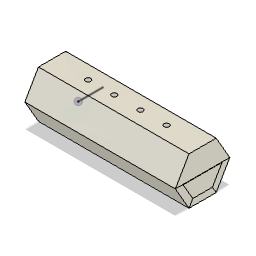
Ares_Pedroli_Dye—Radio (Autodesk Fusion 360 design; units mm, degrees)
Autodesk Fusion 360 part; units mm, degrees
note: some values were not read from the file. Set by a fixed rule: which sketch regions a step uses.
(part 1 of 3)
sketch "Schizzo1" plane through (0, 0, 0) normal (1, 0, 0) x (0, 0, -1)
  line L0 (20.7846, 36) -> (-20.7846, 36)
  line L1 (15.0111, 26) -> (-15.0111, 26)
  line L2 (-15.0111, 26) -> (-20.7846, 36)
  line L3 (15.0111, 26) -> (20.7846, 36)
  dimension "d1" = 36
  dimension "d2" = 26
  measures "d1" distance of origin L0
  measures "d2" distance of origin L1
extrude "Estrusione1" add sketch "Schizzo1" along normal blind 230 contours L0 L1 L2 L3 picked at (5.0037, 32.6667) makes body 1
sketch "Schizzo2" plane through (230, 0, 0) normal (1, 0, 0) x (0, 0, -1)
  line L0 (-15.0111, 26) -> (15.0111, 26)
  line L1 (15.0111, 26) -> (20.7846, 36)
  line L2 (20.7846, 36) -> (-20.7846, 36)
  line L3 (-20.7846, 36) -> (-15.0111, 26)
  line L4 (-15.0111, 26) -> (-20.7846, 36)
  line L5 (-20.7846, 36) -> (-41.5692, 0)
  line L6 (-41.5692, 0) -> (-30.0222, 0)
  line L7 (-30.0222, 0) -> (-15.0111, 26)
  line L8 (-30.0222, 0) -> (-41.5692, 0)
  line L9 (-41.5692, 0) -> (-20.7846, -36)
  line L10 (-20.7846, -36) -> (-15.0111, -26)
  line L11 (-15.0111, -26) -> (-30.0222, 0)
  line L12 (-15.0111, -26) -> (-20.7846, -36)
  line L13 (-20.7846, -36) -> (20.7846, -36)
  line L14 (20.7846, -36) -> (15.0111, -26)
  line L15 (15.0111, -26) -> (-15.0111, -26)
  line L16 (15.0111, -26) -> (20.7846, -36)
  line L17 (20.7846, -36) -> (41.5692, 0)
  line L18 (41.5692, 0) -> (30.0222, 0)
  line L19 (30.0222, 0) -> (15.0111, -26)
  line L20 (30.0222, 0) -> (41.5692, 0)
  line L21 (41.5692, 0) -> (20.7846, 36)
  line L22 (20.7846, 36) -> (15.0111, 26)
  line L23 (15.0111, 26) -> (30.0222, 0)
  dimension "d6" = 360
sketch "Schizzo3" plane through (230, 0, 0) normal (1, 0, 0) x (0, 0, -1)
extrude "Estrusione2" add sketch "Schizzo2" against normal blind 230 separate body contours L3 L4 L5 L6 L7 L8 picked at (-25.7883, 20.6667) makes body 2
sketch "Schizzo4" plane through (230, 0, 0) normal (1, 0, 0) x (0, 0, -1)
  line L0 (-15.0111, 26) -> (15.0111, 26)
  line L1 (15.0111, 26) -> (20.7846, 36)
  line L2 (20.7846, 36) -> (-20.7846, 36)
  line L3 (-20.7846, 36) -> (-15.0111, 26)
  line L4 (-20.7846, 36) -> (-41.5692, 0)
  line L5 (-41.5692, 0) -> (-20.7846, -36)
  line L6 (-20.7846, -36) -> (20.7846, -36)
  line L7 (20.7846, -36) -> (41.5692, 0)
  line L8 (41.5692, 0) -> (20.7846, 36)
  line L9 (20.7846, 36) -> (-20.7846, 36)
  line L10 (-15.0111, 26) -> (-30.0222, 0)
  line L11 (-30.0222, 0) -> (-15.0111, -26)
  line L12 (-15.0111, -26) -> (15.0111, -26)
  line L13 (15.0111, -26) -> (30.0222, 0)
  line L14 (30.0222, 0) -> (15.0111, 26)
  line L15 (15.0111, 26) -> (-15.0111, 26)
  line L16 (-15.0111, -26) -> (-20.7846, -36)
  line L17 (15.0111, -26) -> (20.7846, -36)
  dimension "d9" = 36
  dimension "d10" = 26
  measures "d9" distance of origin L9
  measures "d10" distance of origin L15
extrude "Estrusione3" add sketch "Schizzo4" against normal blind 230 separate body contours L6 L12 L16 L17 picked at (5.0037, -32.6667) makes body 3
sketch "Schizzo5" plane through (230, 0, 0) normal (1, 0, 0) x (0, 0, -1)
  line L0 (-15.0111, 26) -> (-20.7846, 36)
  line L1 (-20.7846, 36) -> (-41.5692, 0)
  line L2 (-41.5692, 0) -> (-30.0222, 0)
  line L3 (-30.0222, 0) -> (-15.0111, 26)
  line L4 (-20.7846, 36) -> (-41.5692, 0)
  line L5 (-41.5692, 0) -> (-20.7846, -36)
  line L6 (-20.7846, -36) -> (20.7846, -36)
  line L7 (20.7846, -36) -> (41.5692, 0)
  line L8 (41.5692, 0) -> (20.7846, 36)
  line L9 (20.7846, 36) -> (-20.7846, 36)
  line L10 (-15.0111, 26) -> (-30.0222, 0)
  line L11 (-30.0222, 0) -> (-15.0111, -26)
  line L12 (-15.0111, -26) -> (15.0111, -26)
  line L13 (15.0111, -26) -> (30.0222, 0)
  line L14 (30.0222, 0) -> (15.0111, 26)
  line L15 (15.0111, 26) -> (-15.0111, 26)
  line L16 (15.0111, -26) -> (20.7846, -36)
  line L17 (30.0222, 0) -> (41.5692, 0)
  dimension "d13" = 36
  dimension "d14" = 26
  constraint horizontal L17
  measures "d13" distance of origin L9
  measures "d14" distance of origin L15
extrude "Estrusione4" add sketch "Schizzo5" against normal blind 230 separate body contours L7 L13 L16 L17 picked at (25.7883, -20.6667) makes body 4
sketch "Schizzo6" plane through (230, 0, 0) normal (1, 0, 0) x (0, 0, -1)
  line L0 (-15.0111, 26) -> (15.0111, 26)
  line L1 (15.0111, 26) -> (20.7846, 36)
  line L2 (20.7846, 36) -> (-20.7846, 36)
  line L3 (-20.7846, 36) -> (-15.0111, 26)
  line L4 (-20.7846, 36) -> (-41.5692, 0)
  line L5 (-41.5692, 0) -> (-20.7846, -36)
  line L6 (-20.7846, -36) -> (20.7846, -36)
  line L7 (20.7846, -36) -> (41.5692, 0)
  line L8 (41.5692, 0) -> (20.7846, 36)
  line L9 (20.7846, 36) -> (-20.7846, 36)
  line L10 (-15.0111, 26) -> (-30.0222, 0)
  line L11 (-30.0222, 0) -> (-15.0111, -26)
  line L12 (-15.0111, -26) -> (15.0111, -26)
  line L13 (15.0111, -26) -> (30.0222, 0)
  line L14 (30.0222, 0) -> (15.0111, 26)
  line L15 (15.0111, 26) -> (-15.0111, 26)
  line L16 (-30.0222, 0) -> (-41.5692, 0)
  line L17 (-15.0111, -26) -> (-20.7846, -36)
  dimension "d17" = 36
  dimension "d18" = 26
  constraint horizontal L16
  measures "d17" distance of origin L9
  measures "d18" distance of origin L15
extrude "Estrusione5" add sketch "Schizzo6" against normal blind 230 separate body contours L5 L11 L16 L17 picked at (-25.7883, -20.6667) makes body 5
sketch "Schizzo7" plane through (230, 0, 0) normal (1, 0, 0) x (0, 0, -1)
  line L0 (-15.0111, 26) -> (15.0111, 26)
  line L1 (15.0111, 26) -> (20.7846, 36)
  line L2 (20.7846, 36) -> (-20.7846, 36)
  line L3 (-20.7846, 36) -> (-15.0111, 26)
  line L4 (-20.7846, 36) -> (-41.5692, 0)
  line L5 (-41.5692, 0) -> (-20.7846, -36)
  line L6 (-20.7846, -36) -> (20.7846, -36)
  line L7 (20.7846, -36) -> (41.5692, 0)
  line L8 (41.5692, 0) -> (20.7846, 36)
  line L9 (20.7846, 36) -> (-20.7846, 36)
  line L10 (-15.0111, 26) -> (-30.0222, 0)
  line L11 (-30.0222, 0) -> (-15.0111, -26)
  line L12 (-15.0111, -26) -> (15.0111, -26)
  line L13 (15.0111, -26) -> (30.0222, 0)
  line L14 (30.0222, 0) -> (15.0111, 26)
  line L15 (15.0111, 26) -> (-15.0111, 26)
  line L16 (30.0222, 0) -> (41.5692, 0)
  line L17 (15.0111, 26) -> (20.7846, 36)
  dimension "d21" = 36
  dimension "d22" = 26
  constraint horizontal L16
  constraint coincident L0.end L1.start
  constraint coincident L1.end L2.start
  measures "d21" distance of origin L9
  measures "d22" distance of origin L15
extrude "Estrusione6" add sketch "Schizzo7" against normal blind 230 separate body contours L1 L8 L14 L16 L17 picked at (25.7883, 20.6667) makes body 6
sketch "Schizzo8" plane through (0, 0, 0) normal (0, -0.5, -0.866025) x (-1, 0, 0)
  line L0 (0, 30.0222) -> (0, 41.5692)
  line L1 (0, 41.5692) -> (-230, 41.5692)
  line L2 (-230, 41.5692) -> (-230, 30.0222)
  line L3 (-230, 30.0222) -> (0, 30.0222)
sketch "Schizzo9" plane through (0, 0, 0) normal (0, -0.5, -0.866025) x (-1, 0, 0)
sketch "Schizzo10" plane through (0, 0, 0) normal (0, 0, 1) x (1, 0, 0)
sketch "Schizzo11" plane through (0, 0, 0) normal (0, 0, 1) x (1, 0, 0)
ref_plane "Piano di lavoro1" through (0, 0, -50) normal (0, 0, 1) x (1, 0, 0)
sketch "Schizzo12" plane through (0, 0, -50) normal (0, 0, 1) x (1, 0, 0)
sketch "Schizzo13" plane through (0, 0, 0) normal (1, 0, 0) x (0, 0, -1)
  line L0 (-20.7846, 36) -> (-41.5692, 0)
  line L1 (-41.5692, 0) -> (-20.7846, -36)
  line L2 (-20.7846, -36) -> (20.7846, -36)
  line L3 (20.7846, -36) -> (41.5692, 0)
  line L4 (41.5692, 0) -> (20.7846, 36)
  line L5 (20.7846, 36) -> (-20.7846, 36)
  dimension "d26" = 36
  measures "d26" distance of origin L5
ref_plane "Piano di lavoro2" through (10, 0, 0) normal (1, 0, 0) x (0, 0, -1)
sketch "Schizzo14" plane through (10, 0, 0) normal (1, 0, 0) x (0, 0, -1)
  line L0 (-15.0111, 26) -> (-30.0222, 0)
  line L1 (-30.0222, 0) -> (-15.0111, -26)
  line L2 (-15.0111, -26) -> (15.0111, -26)
  line L3 (15.0111, -26) -> (30.0222, 0)
  line L4 (30.0222, 0) -> (15.0111, 26)
  line L5 (15.0111, 26) -> (-15.0111, 26)
  dimension "d28" = 26
  measures "d28" distance of origin L5
loft "Loft1" add profiles "Schizzo13", "Schizzo14" section 1 contours L0 L1 L2 L3 L4 L5 picked at (-6.9282, -12) section 2 contours L0 L1 L2 L3 L4 L5 picked at (5.0037, 8.6667) separate body makes body 7
ref_plane "Piano di lavoro3" through (0, 36, 0) normal (0.707107, 0.707107, 0) x (0, 0, 1)
sketch "Schizzo15" plane through (18, 18, 0) normal (0.707107, 0.707107, 0) x (0, 0, 1)
  line L0 (-25.4045, -30.5953) -> (26.5037, -30.5953)
  line L1 (26.5037, -30.5953) -> (26.5037, -11.2977)
  line L2 (26.5037, -11.2977) -> (-25.4045, -11.2977)
  line L3 (-25.4045, -11.2977) -> (-25.4045, -30.5953)
  constraint horizontal L0
  constraint vertical L1
  constraint horizontal L2
  constraint vertical L3
extrude "Estrusione7" cut sketch "Schizzo15" against normal blind 9 contours L0 L1 L2 L3 picked at (9.201, -24.1628) bodies 1
ref_plane "Piano di lavoro4" through (0, -36, 0) normal (-0.707107, 0.707107, 0) x (0, 0, 1)
sketch "Schizzo17" plane through (18, -18, 0) normal (-0.707107, 0.707107, 0) x (0, 0, 1)
  line L0 (-27.9444, 2.5294) -> (34.6896, 2.5294)
  line L1 (34.6896, 2.5294) -> (34.6896, -37.219)
  line L2 (34.6896, -37.219) -> (-27.9444, -37.219)
  line L3 (-27.9444, -37.219) -> (-27.9444, 2.5294)
  constraint horizontal L0
  constraint vertical L1
  constraint horizontal L2
  constraint vertical L3
sketch "Schizzo18" plane through (18, -18, 0) normal (-0.707107, 0.707107, 0) x (0, 0, 1)
extrude "Estrusione8" cut sketch "Schizzo17" along normal blind 15 contours L0 L1 L2 L3 picked at (-7.0664, -10.72) bodies 3
ref_plane "Piano di lavoro5" through (0, 18, -31.1769) normal (0.707107, 0.353553, -0.612372) x (0, -0.866025, -0.5)
sketch "Schizzo19" plane through (18, 9, -15.5885) normal (0.707107, 0.353553, -0.612372) x (0, -0.866025, -0.5)
  line L0 (28.5212, 30.9976) -> (-31.4246, 30.9976)
  line L1 (-31.4246, 30.9976) -> (-31.4246, 0.2562)
  line L2 (-31.4246, 0.2562) -> (28.5212, 0.2562)
  line L3 (28.5212, 0.2562) -> (28.5212, 30.9976)
  constraint horizontal L0
  constraint vertical L1
  constraint horizontal L2
  constraint vertical L3
extrude "Estrusione9" cut sketch "Schizzo19" against normal blind 15 contours L0 L1 L2 L3 picked at (-11.4427, 10.5033) bodies 6
ref_plane "Piano di lavoro6" through (0, -18, 31.1769) normal (0.707107, -0.353553, 0.612372) x (0, 0.866025, 0.5)
sketch "Schizzo20" plane through (18, -9, 15.5885) normal (0.707107, -0.353553, 0.612372) x (0, 0.866025, 0.5)
  line L0 (-39.5033, -4.678) -> (44.909, -4.678)
  line L1 (44.909, -4.678) -> (44.909, 45.013)
  line L2 (44.909, 45.013) -> (-39.5033, 45.013)
  line L3 (-39.5033, 45.013) -> (-39.5033, -4.678)
  constraint horizontal L0
  constraint vertical L1
  constraint horizontal L2
  constraint vertical L3
extrude "Estrusione10" cut sketch "Schizzo20" against normal blind 15 contours L0 L1 L2 L3 picked at (-11.3659, 28.4493) bodies 5
ref_plane "Piano di lavoro7" through (0, 13, 22.5167) normal (0.707107, -0.353553, -0.612372) x (0, -0.866025, 0.5)
sketch "Schizzo21" plane through (-13, 6.5, 11.2583) normal (0.707107, -0.353553, -0.612372) x (0, -0.866025, 0.5)
ref_plane "Piano di lavoro8" through (0, 18, 31.1769) normal (0.707107, 0.353553, 0.612372) x (0, 0.866025, -0.5)
sketch "Schizzo22" plane through (18, 9, 15.5885) normal (0.707107, 0.353553, 0.612372) x (0, 0.866025, -0.5)
  line L0 (34.112, 42.0471) -> (-37.7603, 42.0471)
  line L1 (-37.7603, 42.0471) -> (-37.7603, -13.0428)
  line L2 (-37.7603, -13.0428) -> (34.112, -13.0428)
  line L3 (34.112, -13.0428) -> (34.112, 42.0471)
  constraint horizontal L0
  constraint vertical L1
  constraint horizontal L2
  constraint vertical L3
extrude "Estrusione11" cut sketch "Schizzo22" against normal blind 15 contours L0 L1 L2 L3 picked at (-13.8029, 23.6838) bodies 2
ref_plane "Piano di lavoro9" through (0, -18, -31.1769) normal (0.707107, -0.353553, -0.612372) x (0, -0.866025, 0.5)
sketch "Schizzo23" plane through (18, -9, -15.5885) normal (0.707107, -0.353553, -0.612372) x (0, -0.866025, 0.5)
  line L0 (-34.6034, -9.0564) -> (39.4695, -9.0564)
  line L1 (39.4695, -9.0564) -> (39.4695, 34.7386)
  line L2 (39.4695, 34.7386) -> (-34.6034, 34.7386)
  line L3 (-34.6034, 34.7386) -> (-34.6034, -9.0564)
  constraint horizontal L0
  constraint vertical L1
  constraint horizontal L2
  constraint vertical L3
extrude "Estrusione12" cut sketch "Schizzo23" against normal blind 30 contours L0 L1 L2 L3 picked at (14.7785, 20.1402) bodies 4
sketch "Schizzo24" plane through (230, 0, 0) normal (1, 0, 0) x (0, 0, -1)
  line L0 (-15.0111, 26) -> (15.0111, 26)
  line L1 (15.0111, 26) -> (20.7846, 36)
  line L2 (20.7846, 36) -> (-20.7846, 36)
  line L3 (-20.7846, 36) -> (-15.0111, 26)
  line L4 (-20.7846, 36) -> (-41.5692, 0)
  line L5 (-41.5692, 0) -> (-20.7846, -36)
  line L6 (-20.7846, -36) -> (20.7846, -36)
  line L7 (20.7846, -36) -> (41.5692, 0)
  line L8 (41.5692, 0) -> (20.7846, 36)
  line L9 (20.7846, 36) -> (-20.7846, 36)
  dimension "d48" = 36
  measures "d48" distance of origin L9
ref_plane "Piano di lavoro10" through (220, 0, 0) normal (1, 0, 0) x (0, 0, -1)
sketch "Schizzo25" plane through (220, 0, 0) normal (1, 0, 0) x (0, 0, -1)
  line L0 (-15.0111, 26) -> (-30.0222, 0)
  line L1 (-30.0222, 0) -> (-15.0111, -26)
  line L2 (-15.0111, -26) -> (15.0111, -26)
  line L3 (15.0111, -26) -> (30.0222, 0)
  line L4 (30.0222, 0) -> (15.0111, 26)
  line L5 (15.0111, 26) -> (-15.0111, 26)
  dimension "d50" = 26
  measures "d50" distance of origin L5
loft "Loft2" add profiles "Schizzo24", "Schizzo25" section 1 contours L0 L1 L2 L3 L9 | L0 L1 L3 L4 L5 L6 L7 L8 picked at (5.0037, 32.6667) picked at (5.0037, -15.3333) section 2 contours L0 L1 L2 L3 L4 L5 picked at (5.0037, 8.6667) separate body makes body 8
sketch "Schizzo26" plane through (230, 0, 0) normal (1, 0, 0) x (0, 0, -1)
  line L0 (-15.0111, 26) -> (15.0111, 26)
  line L1 (15.0111, 26) -> (20.7846, 36)
  line L2 (20.7846, 36) -> (-20.7846, 36)
  line L3 (-20.7846, 36) -> (-15.0111, 26)
ref_plane "Piano di lavoro11" through (230, 31, 0) normal (1, 0, 0) x (0, 0, -1)
ref_plane "Piano di lavoro12" through (230, 18, 31.1769) normal (0.707107, -0.353553, -0.612372) x (0, -0.866025, 0.5)
sketch "Schizzo27" plane through (97, -48.5, -84.0045) normal (0.707107, -0.353553, -0.612372) x (0, -0.866025, 0.5)
  line L0 (22.2001, -191.6814) -> (-22.8191, -191.6814)
  line L1 (-22.8191, -191.6814) -> (-22.8191, -156.9019)
  line L2 (-22.8191, -156.9019) -> (22.2001, -156.9019)
  line L3 (22.2001, -156.9019) -> (22.2001, -191.6814)
  constraint horizontal L0
  constraint vertical L1
  constraint horizontal L2
  constraint vertical L3
extrude "Estrusione13" cut sketch "Schizzo27" along normal blind 15 contours L0 L1 L2 L3 picked at (7.1937, -168.495) bodies 2
ref_plane "Piano di lavoro13" through (230, 36, 0) normal (-0.707107, 0.707107, 0) x (0, 0, 1)
sketch "Schizzo28" plane through (97, -97, 0) normal (-0.707107, 0.707107, 0) x (0, 0, 1)
  line L0 (24.2107, 192.65) -> (-25.7482, 192.65)
  line L1 (-25.7482, 192.65) -> (-25.7482, 160.1447)
  line L2 (-25.7482, 160.1447) -> (24.2107, 160.1447)
  line L3 (24.2107, 160.1447) -> (24.2107, 192.65)
  constraint horizontal L0
  constraint vertical L1
  constraint horizontal L2
  constraint vertical L3
extrude "Estrusione14" cut sketch "Schizzo28" against normal blind 15 contours L0 L1 L2 L3 picked at (-9.0953, 181.8149) bodies 1
ref_plane "Piano di lavoro14" through (230, 18, -31.1769) normal (0.707107, -0.353553, 0.612372) x (0, 0.866025, 0.5)
sketch "Schizzo29" plane through (97, -48.5, 84.0045) normal (0.707107, -0.353553, 0.612372) x (0, 0.866025, 0.5)
  line L0 (24.9926, -195.9491) -> (-24.9663, -195.9491)
  line L1 (-24.9663, -195.9491) -> (-24.9663, -159.7609)
  line L2 (-24.9663, -159.7609) -> (24.9926, -159.7609)
  line L3 (24.9926, -159.7609) -> (24.9926, -195.9491)
  constraint horizontal L0
  constraint vertical L1
  constraint horizontal L2
  constraint vertical L3
extrude "Estrusione15" cut sketch "Schizzo29" along normal blind 15 contours L0 L1 L2 L3 picked at (8.3396, -183.8864) bodies 6
sketch "Schizzo30" plane through (230, 0, 0) normal (1, 0, 0) x (0, 0, -1)
  line L0 (20.7846, 36) -> (-20.7846, 36)
  line L1 (-20.7846, 36) -> (-41.5692, 0)
  line L2 (-41.5692, 0) -> (-20.7846, -36)
  line L3 (-20.7846, -36) -> (20.7846, -36)
  line L4 (20.7846, -36) -> (41.5692, 0)
  line L5 (41.5692, 0) -> (20.7846, 36)
  line L6 (-51.0641, 0) -> (47.9858, 0)
  line L7 (47.9858, 0) -> (47.9858, -40.8332)
  line L8 (47.9858, -40.8332) -> (-51.0641, -40.8332)
  line L9 (-51.0641, -40.8332) -> (-51.0641, 0)
  constraint horizontal L6
  constraint vertical L7
  constraint horizontal L8
  constraint vertical L9
extrude "Estrusione16" cut sketch "Schizzo30" against normal blind 50 contours L2 L3 L4 L6 L7 L8 L9 | L2 L3 L4 L6 picked at (-37.806, -25.6111) picked at (-6.9282, -12) bodies 8
sketch "Schizzo31" plane through (0, 0, 0) normal (1, 0, 0) x (0, 0, -1)
ref_plane "Piano di lavoro15" through (230, 0, 0) normal (1, 0, 0) x (0, 1, 0)
sketch "Schizzo32" plane through (230, 0, 0) normal (1, 0, 0) x (0, 0, -1)
  line L0 (-15.0111, 26) -> (-30.0222, 0)
  line L1 (-30.0222, 0) -> (-15.0111, -26)
  line L2 (-15.0111, -26) -> (15.0111, -26)
  line L3 (15.0111, -26) -> (30.0222, 0)
  line L4 (30.0222, 0) -> (15.0111, 26)
  line L5 (15.0111, 26) -> (-15.0111, 26)
  line L6 (-12.1244, 21) -> (-24.2487, 0)
  line L7 (-24.2487, 0) -> (-12.1244, -21)
  line L8 (-12.1244, -21) -> (12.1244, -21)
  line L9 (12.1244, -21) -> (24.2487, 0)
  line L10 (24.2487, 0) -> (12.1244, 21)
  line L11 (12.1244, 21) -> (-12.1244, 21)
  line L12 (-24.2487, 0) -> (-30.0222, 0)
  line L13 (-12.1244, -21) -> (-15.0111, -26)
  dimension "d64" = 26
  dimension "d65" = 21
  constraint horizontal L12
  measures "d64" distance of origin L5
  measures "d65" distance of origin L11
extrude "Estrusione17" add sketch "Schizzo32" against normal blind 190 separate body contours L1 L7 L12 L13 picked at (-19.0526, -15.6667) makes body 9
sketch "Schizzo33" plane through (230, 0, 0) normal (1, 0, 0) x (0, 0, -1)
  line L0 (-24.2487, 0) -> (-30.0222, 0)
  line L1 (-30.0222, 0) -> (-15.0111, -26)
  line L2 (-15.0111, -26) -> (-12.1244, -21)
  line L3 (-12.1244, -21) -> (-24.2487, 0)
  line L4 (-15.0111, 26) -> (-30.0222, 0)
  line L5 (-30.0222, 0) -> (-15.0111, -26)
  line L6 (-15.0111, -26) -> (15.0111, -26)
  line L7 (15.0111, -26) -> (30.0222, 0)
  line L8 (30.0222, 0) -> (15.0111, 26)
  line L9 (15.0111, 26) -> (-15.0111, 26)
  line L10 (12.1244, -21) -> (24.2487, 0)
  line L11 (24.2487, 0) -> (12.1244, 21)
  line L12 (12.1244, 21) -> (-12.1244, 21)
  line L13 (-12.1244, 21) -> (-24.2487, 0)
  line L14 (-24.2487, 0) -> (-12.1244, -21)
  line L15 (-12.1244, -21) -> (12.1244, -21)
  line L16 (12.1244, -21) -> (15.0111, -26)
  line L17 (24.2487, 0) -> (30.0222, 0)
  dimension "d68" = 26
  dimension "d69" = 21
  constraint horizontal L17
  measures "d68" distance of origin L9
  measures "d69" distance of origin L15
extrude "Estrusione18" add sketch "Schizzo33" against normal blind 190 separate body contours L7 L10 L16 L17 picked at (19.0526, -15.6667) makes body 10
sketch "Schizzo34" plane through (230, 0, 0) normal (1, 0, 0) x (0, 0, -1)
  line L0 (-24.2487, 0) -> (-30.0222, 0)
  line L1 (-30.0222, 0) -> (-15.0111, -26)
  line L2 (-15.0111, -26) -> (-12.1244, -21)
  line L3 (-12.1244, -21) -> (-24.2487, 0)
  line L4 (-15.0111, 26) -> (-30.0222, 0)
  line L5 (-30.0222, 0) -> (-15.0111, -26)
  line L6 (-15.0111, -26) -> (15.0111, -26)
  line L7 (15.0111, -26) -> (30.0222, 0)
  line L8 (30.0222, 0) -> (15.0111, 26)
  line L9 (15.0111, 26) -> (-15.0111, 26)
  line L10 (12.1244, -21) -> (24.2487, 0)
  line L11 (24.2487, 0) -> (12.1244, 21)
  line L12 (12.1244, 21) -> (-12.1244, 21)
  line L13 (-12.1244, 21) -> (-24.2487, 0)
  line L14 (-24.2487, 0) -> (-12.1244, -21)
  line L15 (-12.1244, -21) -> (12.1244, -21)
  line L16 (-12.1244, -21) -> (-15.0111, -26)
  line L17 (12.1244, -21) -> (15.0111, -26)
  dimension "d72" = 26
  dimension "d73" = 21
  constraint coincident L2.end L3.start
  constraint parallel L2 L16
  measures "d72" distance of origin L9
  measures "d73" distance of origin L15
extrude "Estrusione19" add sketch "Schizzo34" against normal blind 190 separate body contours L2 L6 L15 L16 L17 picked at (4.0415, -24.3333) makes body 11
sketch "Schizzo35" plane through (230, 0, 0) normal (1, 0, 0) x (0, 0, -1)
  line L0 (-12.1244, -21) -> (-15.0111, -26)
  line L1 (-15.0111, -26) -> (15.0111, -26)
  line L2 (15.0111, -26) -> (12.1244, -21)
  line L3 (12.1244, -21) -> (-12.1244, -21)
  line L4 (-15.0111, 26) -> (-30.0222, 0)
  line L5 (-30.0222, 0) -> (-15.0111, -26)
  line L6 (-15.0111, -26) -> (15.0111, -26)
  line L7 (15.0111, -26) -> (30.0222, 0)
  line L8 (30.0222, 0) -> (15.0111, 26)
  line L9 (15.0111, 26) -> (-15.0111, 26)
  dimension "d76" = 26
  measures "d76" distance of origin L9
ref_plane "Piano di lavoro16" through (225, 0, 0) normal (1, 0, 0) x (0, 0, -1)
sketch "Schizzo36" plane through (230, 0, 0) normal (1, 0, 0) x (0, 0, -1)
  line L0 (-41.5692, 0) -> (41.5692, 0)
  line L1 (41.5692, 0) -> (20.7846, 36)
  line L2 (20.7846, 36) -> (-20.7846, 36)
  line L3 (-20.7846, 36) -> (-41.5692, 0)
  line L4 (-15.0111, 26) -> (-30.0222, 0)
  line L5 (-30.0222, 0) -> (-15.0111, -26)
  line L6 (-15.0111, -26) -> (15.0111, -26)
  line L7 (15.0111, -26) -> (30.0222, 0)
  line L8 (30.0222, 0) -> (15.0111, 26)
  line L9 (15.0111, 26) -> (-15.0111, 26)
  dimension "d78" = 26
  measures "d78" distance of origin L9
sketch "Schizzo37" plane through (225, 0, 0) normal (1, 0, 0) x (0, 0, -1)
  line L0 (-12.1244, 21) -> (-24.2487, 0)
  line L1 (-24.2487, 0) -> (-12.1244, -21)
  line L2 (-12.1244, -21) -> (12.1244, -21)
  line L3 (12.1244, -21) -> (24.2487, 0)
  line L4 (24.2487, 0) -> (12.1244, 21)
  line L5 (12.1244, 21) -> (-12.1244, 21)
  dimension "d79" = 21
  measures "d79" distance of origin L5
loft "Loft3" add profiles "Schizzo35", "Schizzo37" section 1 contours L0 L1 L2 L3 L6 | L0 L2 L3 L4 L5 L7 L8 L9 picked at (4.0415, -24.3333) picked at (-4.0415, 10.3333) section 2 contours L0 L1 L2 L3 L4 L5 picked at (4.0415, 7) separate body makes body 12
ref_plane "Piano di lavoro17" through (230, -26, 0) normal (0.707107, 0.707107, 0) x (0, 0, -1)
sketch "Schizzo38" plane through (102, 102, 0) normal (0.707107, 0.707107, 0) x (0, 0, -1)
  line L0 (-16.091, -182.4296) -> (16.5053, -182.4296)
  line L1 (16.5053, -182.4296) -> (16.5053, -162.3983)
  line L2 (16.5053, -162.3983) -> (-16.091, -162.3983)
  line L3 (-16.091, -162.3983) -> (-16.091, -182.4296)
  constraint horizontal L0
  constraint vertical L1
  constraint horizontal L2
  constraint vertical L3
extrude "Estrusione20" cut sketch "Schizzo38" along normal blind 6 contours L0 L1 L2 L3 picked at (-5.2256, -169.0754) bodies 11
ref_plane "Piano di lavoro18" through (230, -13, -22.5167) normal (0.707107, 0.353553, 0.612372) x (0, 0.866025, -0.5)
sketch "Schizzo39" plane through (102, 51, 88.3346) normal (0.707107, 0.353553, 0.612372) x (0, 0.866025, -0.5)
  line L0 (-15.7064, -182.521) -> (18.7477, -182.521)
  line L1 (18.7477, -182.521) -> (18.7477, -158.8555)
  line L2 (18.7477, -158.8555) -> (-15.7064, -158.8555)
  line L3 (-15.7064, -158.8555) -> (-15.7064, -182.521)
  constraint horizontal L0
  constraint vertical L1
  constraint horizontal L2
  constraint vertical L3
sketch "Schizzo40" plane through (102, 51, 88.3346) normal (0.707107, 0.353553, 0.612372) x (0, 0.866025, -0.5)
extrude "Estrusione21" cut sketch "Schizzo39" along normal blind 7 contours L0 L1 L2 L3 picked at (-4.2217, -174.6325) bodies 10
ref_plane "Piano di lavoro19" through (230, -13, 22.5167) normal (0.707107, 0.353553, -0.612372) x (0, -0.866025, -0.5)
sketch "Schizzo41" plane through (102, 51, -88.3346) normal (0.707107, 0.353553, -0.612372) x (0, -0.866025, -0.5)
  line L0 (-15.9646, -162.8849) -> (17.7885, -162.8849)
  line L1 (17.7885, -162.8849) -> (17.7885, -184.9057)
  line L2 (17.7885, -184.9057) -> (-15.9646, -184.9057)
  line L3 (-15.9646, -184.9057) -> (-15.9646, -162.8849)
  constraint horizontal L0
  constraint vertical L1
  constraint horizontal L2
  constraint vertical L3
extrude "Estrusione22" cut sketch "Schizzo41" along normal blind 5 contours L0 L1 L2 L3 picked at (-4.7135, -170.2252) bodies 9
sketch "Schizzo42" plane through (230, 0, 0) normal (1, 0, 0) x (0, 0, -1)
  line L0 (15.0111, 26) -> (-15.0111, 26)
  line L1 (-15.0111, 26) -> (-30.0222, 0)
  line L2 (-30.0222, 0) -> (-15.0111, -26)
  line L3 (-15.0111, -26) -> (15.0111, -26)
  line L4 (15.0111, -26) -> (30.0222, 0)
  line L5 (30.0222, 0) -> (15.0111, 26)
  line L6 (-35.3311, 0) -> (32.3333, 0)
  line L7 (32.3333, 0) -> (32.3333, 27.8901)
  line L8 (32.3333, 27.8901) -> (-35.3311, 27.8901)
  line L9 (-35.3311, 27.8901) -> (-35.3311, 0)
  constraint horizontal L6
  constraint vertical L7
  constraint horizontal L8
  constraint vertical L9
extrude "Estrusione23" cut sketch "Schizzo42" against normal blind 11 contours L0 L1 L5 L6 | L0 L1 L5 L6 L7 L8 L9 picked at (5.0037, 8.6667) picked at (-26.7881, 17.9634) bodies 12
ref_plane "Piano di lavoro20" through (40, -13, -22.5167) normal (0.707107, -0.353553, -0.612372) x (0, -0.866025, 0.5)
sketch "Schizzo43" plane through (33, -16.5, -28.5788) normal (0.707107, -0.353553, -0.612372) x (0, -0.866025, 0.5)
  line L0 (-15.7171, -8.5355) -> (17.9237, -8.5355)
  line L1 (17.9237, -8.5355) -> (17.9237, -25.9435)
  line L2 (17.9237, -25.9435) -> (-15.7171, -25.9435)
  line L3 (-15.7171, -25.9435) -> (-15.7171, -8.5355)
  constraint horizontal L0
  constraint vertical L1
  constraint horizontal L2
  constraint vertical L3
extrude "Estrusione24" cut sketch "Schizzo43" against normal blind 6 contours L0 L1 L2 L3 picked at (-4.5035, -14.3381) bodies 10
ref_plane "Piano di lavoro21" through (40, -26, 0) normal (-0.707107, 0.707107, 0) x (0, 0, 1)
sketch "Schizzo44" plane through (33, -33, 0) normal (-0.707107, 0.707107, 0) x (0, 0, 1)
  line L0 (-17.0445, 8.6761) -> (20.7303, 8.6761)
  line L1 (20.7303, 8.6761) -> (20.7303, 23.9726)
  line L2 (20.7303, 23.9726) -> (-17.0445, 23.9726)
  line L3 (-17.0445, 23.9726) -> (-17.0445, 8.6761)
  constraint horizontal L0
  constraint vertical L1
  constraint horizontal L2
  constraint vertical L3
extrude "Estrusione25" cut sketch "Schizzo44" along normal blind 8 contours L0 L1 L2 L3 picked at (-4.4529, 13.775) bodies 11
ref_plane "Piano di lavoro22" through (40, -13, 22.5167) normal (0.707107, -0.353553, 0.612372) x (0, 0.866025, 0.5)
sketch "Schizzo45" plane through (33, -16.5, 28.5788) normal (0.707107, -0.353553, 0.612372) x (0, 0.866025, 0.5)
  line L0 (-16.1058, -7.4381) -> (17.3139, -7.4381)
  line L1 (17.3139, -7.4381) -> (17.3139, -25.1355)
  line L2 (17.3139, -25.1355) -> (-16.1058, -25.1355)
  line L3 (-16.1058, -25.1355) -> (-16.1058, -7.4381)
  constraint horizontal L0
  constraint vertical L1
  constraint horizontal L2
  constraint vertical L3
extrude "Estrusione26" cut sketch "Schizzo45" against normal blind 7 contours L0 L1 L2 L3 picked at (-4.9659, -13.3372) bodies 9
ref_plane "Piano di lavoro23" through (40, 0, 0) normal (1, 0, 0) x (0, 1, 0)
sketch "Schizzo46" plane through (40, 0, 0) normal (1, 0, 0) x (0, 0, -1)
  line L0 (-15.0111, 26) -> (-30.0222, 0)
  line L1 (-30.0222, 0) -> (-15.0111, -26)
  line L2 (-15.0111, -26) -> (15.0111, -26)
  line L3 (15.0111, -26) -> (30.0222, 0)
  line L4 (30.0222, 0) -> (15.0111, 26)
  line L5 (15.0111, 26) -> (-15.0111, 26)
  dimension "d101" = 26
  measures "d101" distance of origin L5
ref_plane "Piano di lavoro24" through (45, 0, 0) normal (1, 0, 0) x (0, 0, -1)
sketch "Schizzo47" plane through (45, 0, 0) normal (1, 0, 0) x (0, 0, -1)
  line L0 (-12.1244, 21) -> (-24.2487, 0)
  line L1 (-24.2487, 0) -> (-12.1244, -21)
  line L2 (-12.1244, -21) -> (12.1244, -21)
  line L3 (12.1244, -21) -> (24.2487, 0)
  line L4 (24.2487, 0) -> (12.1244, 21)
  line L5 (12.1244, 21) -> (-12.1244, 21)
  dimension "d103" = 21
  measures "d103" distance of origin L5
loft "Loft4" add profiles "Schizzo46", "Schizzo47" section 1 contours L0 L1 L2 L3 L4 L5 picked at (-5.0037, -8.6667) section 2 contours L0 L1 L2 L3 L4 L5 picked at (-4.0415, 7) separate body makes body 13
sketch "Schizzo48" plane through (40, 0, 0) normal (-1, 0, 0) x (0, 0, 1)
  line L0 (15.0111, 26) -> (-15.0111, 26)
  line L1 (-15.0111, 26) -> (-30.0222, 0)
  line L2 (-30.0222, 0) -> (-15.0111, -26)
  line L3 (-15.0111, -26) -> (15.0111, -26)
  line L4 (15.0111, -26) -> (30.0222, 0)
  line L5 (30.0222, 0) -> (15.0111, 26)
  line L6 (-38.2161, 0) -> (38.5243, 0)
  line L7 (38.5243, 0) -> (38.5243, 31.2047)
  line L8 (38.5243, 31.2047) -> (-38.2161, 31.2047)
  line L9 (-38.2161, 31.2047) -> (-38.2161, 0)
  constraint horizontal L6
  constraint vertical L7
  constraint horizontal L8
  constraint vertical L9
sketch "Schizzo49" plane through (40, 0, 0) normal (-1, 0, 0) x (0, 0, 1)
extrude "Estrusione27" cut sketch "Schizzo48" against normal blind 10 contours L0 L1 L5 L6 | L0 L1 L5 L6 L7 L8 L9 picked at (5.0037, 8.6667) picked at (27.8526, 19.0682) bodies 13
sketch "Schizzo50" plane through (0, 0, 0) normal (1, 0, 0) x (0, 0, -1)
sketch "Schizzo51" plane through (0, 0, 0) normal (1, 0, 0) x (0, 0, -1)
ref_plane "Piano di lavoro25" through (40, 0, 0) normal (-1, 0, 0) x (0, 0, 1)
sketch "Schizzo54" plane through (40, 0, 0) normal (-1, 0, 0) x (0, 0, 1)
  line L0 (30.0222, 0) -> (-30.0222, 0)
  line L1 (-30.0222, 0) -> (-15.0111, -26)
  line L2 (-15.0111, -26) -> (15.0111, -26)
  line L3 (15.0111, -26) -> (30.0222, 0)
  line L4 (-33.5294, 0) -> (36.4092, 0)
  line L5 (36.4092, 0) -> (36.4092, -0.5)
  line L6 (36.4092, -0.5) -> (-33.5294, -0.5)
  line L7 (-33.5294, -0.5) -> (-33.5294, 0)
  dimension "d114" = 0.5
  constraint horizontal L4
  constraint vertical L5
  constraint horizontal L6
  constraint vertical L7
  measures "d114" distance of L4.start L6.end
sketch "Schizzo55" plane through (40, 0, 0) normal (-1, 0, 0) x (0, 0, 1)
extrude "Estrusione30" cut sketch "Schizzo54" against normal blind 10 contours L0 L1 L3 L4 L6 picked at (9.9112, -0.1667) bodies 13
sketch "Schizzo56" plane through (40, 0, 0) normal (-1, 0, 0) x (0, 0, 1)
  line L0 (29.7335, -0.5) -> (-29.7335, -0.5)
  line L1 (-29.7335, -0.5) -> (-15.0111, -26)
  line L2 (-15.0111, -26) -> (15.0111, -26)
  line L3 (15.0111, -26) -> (29.7335, -0.5)
  line L4 (0, 0) -> (47.3428, 0)
  line L5 (47.3428, 0) -> (47.3428, -0.5)
  line L6 (47.3428, -0.5) -> (0, -0.5)
  line L7 (0, -0.5) -> (0, 0)
  dimension "d117" = 0.5
  constraint horizontal L4
  constraint vertical L5
  constraint horizontal L6
  constraint vertical L7
  constraint coincident L4.start L7.end
  measures "d117" distance of L4.start L6.end
extrude "Estrusione31" cut sketch "Schizzo56" against normal blind 205 contours L0 L4 L5 L6 L7 picked at (25.6921, -0.1667) bodies 9
sketch "Schizzo57" plane through (40, 0, 0) normal (-1, 0, 0) x (0, 0, 1)
  line L0 (29.7335, -0.5) -> (-29.7335, -0.5)
  line L1 (-29.7335, -0.5) -> (-15.0111, -26)
  line L2 (-15.0111, -26) -> (15.0111, -26)
  line L3 (15.0111, -26) -> (29.7335, -0.5)
  line L4 (0, 0) -> (-37.4652, 0)
  line L5 (-37.4652, 0) -> (-37.4652, -0.5)
  line L6 (-37.4652, -0.5) -> (0, -0.5)
  line L7 (0, -0.5) -> (0, 0)
  dimension "d120" = 0.5
  constraint horizontal L4
  constraint vertical L5
  constraint horizontal L6
  constraint vertical L7
  constraint coincident L4.start L7.end
  measures "d120" distance of L4.start L6.end
extrude "Estrusione32" cut sketch "Schizzo57" against normal blind 198 contours L0 L4 L5 L6 L7 picked at (-22.3996, -0.1667) bodies 10
sketch "Schizzo58" plane through (40, 0, 0) normal (-1, 0, 0) x (0, 0, 1)
  line L0 (29.7335, -0.5) -> (-29.7335, -0.5)
  line L1 (-29.7335, -0.5) -> (-15.0111, -26)
  line L2 (-15.0111, -26) -> (15.0111, -26)
  line L3 (15.0111, -26) -> (29.7335, -0.5)
  line L4 (-32.6364, 0) -> (33.0455, 0)
  line L5 (33.0455, 0) -> (33.0455, -0.5)
  line L6 (33.0455, -0.5) -> (-32.6364, -0.5)
  line L7 (-32.6364, -0.5) -> (-32.6364, 0)
  dimension "d123" = 0.5
  constraint horizontal L4
  constraint vertical L5
  constraint horizontal L6
  constraint vertical L7
  measures "d123" distance of L4.start L6.end
extrude "Estrusione33" cut sketch "Schizzo58" against normal blind 210 contours L0 L4 L5 L6 L7 picked at (-9.7748, -0.1667) bodies 12
sketch "Schizzo59" plane through (230, 0, 0) normal (1, 0, 0) x (0, 0, -1)
sketch "Schizzo61" plane through (0, 0, 0) normal (-1, 0, 0) x (0, 0, 1)
  line L0 (20.7846, 36) -> (-20.7846, 36)
  line L1 (-20.7846, 36) -> (-41.5692, 0)
  line L2 (-41.5692, 0) -> (-20.7846, -36)
  line L3 (-20.7846, -36) -> (20.7846, -36)
  line L4 (20.7846, -36) -> (41.5692, 0)
  line L5 (41.5692, 0) -> (20.7846, 36)
  circle A0 centre (0, 0) radius 3
  dimension "d132" = 6
  constraint coincident A0.centre origin
  measures "d132" diameter of A0
extrude "Estrusione35" cut sketch "Schizzo61" against normal blind 10 contours A0 picked at (-1.1591, 0.5829) bodies 7
sketch "Schizzo62" plane through (0, -26, 0) normal (0, 1, 0) x (-1, 0, 0)
  line L0 (-10, -15.0111) -> (-10, 15.0111)
  line L1 (-10, 15.0111) -> (-230, 15.0111)
  line L2 (-230, 15.0111) -> (-230, -15.0111)
  line L3 (-230, -15.0111) -> (-10, -15.0111)
  circle A0 centre (-20.0339, 0) radius 4
  dimension "d135" = 8
  measures "d135" diameter of A0
extrude "Estrusione36" cut sketch "Schizzo62" against normal blind 12 contours A0 picked at (-21.0377, -2.1865) bodies 3
sketch "Schizzo63" plane through (0, 26, 0) normal (0, -1, 0) x (1, 0, 0)
  line L0 (220, -15.0111) -> (220, 15.0111)
  line L1 (220, 15.0111) -> (10, 15.0111)
  line L2 (10, 15.0111) -> (10, -15.0111)
  line L3 (10, -15.0111) -> (220, -15.0111)
  line L4 (0, 0) -> (55, 0)
  dimension "d138" = 55
  constraint coincident L4.start origin
  constraint horizontal L4
  measures "d138" distance of L4.start L4.end
hole "Foratura1" at (55, 26, 0) direction (0, 1, 0) diameter 8 depth 15 tip angle 118 bodies 1
sketch "Schizzo64" plane through (0, 26, 0) normal (0, -1, 0) x (1, 0, 0)
  circle A0 centre (55, 0) radius 4
  line L0 (220, -15.0111) -> (220, 15.0111)
  line L1 (220, 15.0111) -> (10, 15.0111)
  line L2 (10, 15.0111) -> (10, -15.0111)
  line L3 (10, -15.0111) -> (220, -15.0111)
sketch "Schizzo65" plane through (0, 26, 0) normal (0, -1, 0) x (1, 0, 0)
  line L0 (0, 0) -> (95, 0)
  circle A0 centre (95, 0) radius 4
  dimension "d142" = 95
  dimension "d143" = 8
  constraint coincident L0.start origin
  constraint horizontal L0
  constraint coincident L0.end A0.centre
  measures "d142" distance of L0.start L0.end
  measures "d143" diameter of A0
extrude "Estrusione37" cut sketch "Schizzo65" against normal blind 15 contours A0 picked at (92.7042, 1.1056) bodies 1
sketch "Schizzo66" plane through (0, 26, 0) normal (0, -1, 0) x (1, 0, 0)
  line L0 (0, 0) -> (135, 0)
  circle A0 centre (135, 0) radius 4
  dimension "d146" = 135
  dimension "d147" = 8
  constraint coincident L0.start origin
  constraint horizontal L0
  constraint coincident L0.end A0.centre
  measures "d146" distance of L0.start L0.end
  measures "d147" diameter of A0
extrude "Estrusione38" cut sketch "Schizzo66" against normal blind 20 contours A0 picked at (137.1054, -1.1644) bodies 1
sketch "Schizzo67" plane through (0, 26, 0) normal (0, -1, 0) x (1, 0, 0)
  line L0 (0, 0) -> (175, 0)
  circle A0 centre (175, 0) radius 4
  dimension "d150" = 175
  dimension "d151" = 8
  constraint coincident L0.start origin
  constraint horizontal L0
  constraint coincident L0.end A0.centre
  measures "d150" distance of L0.start L0.end
  measures "d151" diameter of A0
extrude "Estrusione39" cut sketch "Schizzo67" against normal blind 20 contours A0 picked at (177.1054, -1.1644) bodies 1
sketch "Schizzo68" plane through (0, 0, 0) normal (1, 0, 0) x (0, 0, -1)
sketch "Schizzo69" plane through (0, 0, 0) normal (-1, 0, 0) x (0, 0, 1)
  circle A0 centre (0, 0) radius 3
  line L0 (20.7846, 36) -> (-20.7846, 36)
  line L1 (-20.7846, 36) -> (-41.5692, 0)
  line L2 (-41.5692, 0) -> (-20.7846, -36)
  line L3 (-20.7846, -36) -> (20.7846, -36)
  line L4 (20.7846, -36) -> (41.5692, 0)
  line L5 (41.5692, 0) -> (20.7846, 36)
sketch "Schizzo70" plane through (0, 0, 0) normal (0, 0, 1) x (1, 0, 0)
sketch "Schizzo71" plane through (0, 0, 0) normal (-1, 0, 0) x (0, 0, 1)
  line L0 (-7.2169, 12.5) -> (-14.4338, 0)
  line L1 (-14.4338, 0) -> (-7.2169, -12.5)
  line L2 (-7.2169, -12.5) -> (7.2169, -12.5)
  line L3 (7.2169, -12.5) -> (14.4338, 0)
  line L4 (14.4338, 0) -> (7.2169, 12.5)
  line L5 (7.2169, 12.5) -> (-7.2169, 12.5)
  dimension "d154" = 12.5
  measures "d154" distance of origin L5
extrude "Estrusione40" add sketch "Schizzo71" along normal blind 7 separate body contours L0 L1 L2 L3 L4 L5 picked at (2.4056, 4.1667) makes body 14
sketch "Schizzo72" plane through (0, -36, 0) normal (0, -1, 0) x (1, 0, 0)
  circle A0 centre (20.0339, 0) radius 4
  line L0 (230, -20.7846) -> (230, 20.7846)
  line L1 (230, 20.7846) -> (0, 20.7846)
  line L2 (0, 20.7846) -> (0, -20.7846)
  line L3 (0, -20.7846) -> (230, -20.7846)
  line L4 (230, 0) -> (210, 0)
  line L5 (210, 0) -> (190, 0)
  circle A1 centre (190, 0) radius 10
  line L6 (190.0034, 10) -> (160.0034, 10)
  line L7 (160.0034, 10) -> (160.0034, -10)
  line L8 (160.0034, -10) -> (190.0034, -10)
  line L9 (190.0034, -10) -> (190.0034, 10)
  circle A2 centre (160.0034, 0) radius 10
  dimension "d157" = 20
  dimension "d158" = 20
  dimension "d159" = 20
  dimension "d160" = 30
  dimension "d161" = 20
  dimension "d162" = 20
  constraint midpoint L0 L4.start
  constraint perpendicular L0 L4
  constraint parallel L4 L5
  constraint coincident L5.end A1.centre
  constraint horizontal L6
  constraint vertical L7
  constraint horizontal L8
  constraint vertical L9
  constraint coincident A1 L6.start
  constraint midpoint L7 A2.centre
  measures "d157" distance of L4.start L4.end
  measures "d158" distance of L4.end L5.end
  measures "d159" diameter of A1
  measures "d160" distance of L6.start L6.end
  measures "d161" distance of L6.start L8.end
  measures "d162" diameter of A2
extrude "Estrusione41" cut sketch "Schizzo72" against normal blind 10 contours L5 A1 L9 | L5 A1 L9 | A1 L9 | L7 A2 | L7 A2 picked at (190.4765, -6.6326) picked at (191.4165, 6.4973) picked at (189.5065, -6.6296) picked at (166.7693, -1.4521) picked at (156.6794, 0.2491) bodies 3
sketch "Schizzo73" plane through (97, -48.5, 84.0045) normal (-0.707107, 0.353553, -0.612372) x (-0.654654, 0, 0.755929)
  line L0 (-166.282, 90.3343) -> (-181.9937, 51.8487)
  line L1 (-181.9937, 51.8487) -> (-166.7185, 51.8487)
  line L2 (-166.7185, 51.8487) -> (-155.3711, 79.6439)
  line L3 (-155.3711, 79.6439) -> (-166.282, 90.3343)
sketch "Schizzo74" plane through (0, 0, 0) normal (0, 0, 1) x (1, 0, 0)
move_body "Sposta5" bodies 14 to x (1, 0, 0) y (0, 1, 0) z (0, 0, 1) at (-1, 0, 0)
sketch "Schizzo87" plane through (0, -26, 0) normal (0, 1, 0) x (-1, 0, 0)
  arc A0 (-160.0034, -10) -> (-160.0034, 10) centre (-160.0034, 0) ccw
  line L0 (-160.0034, -10) -> (-190.0034, -10)
  arc A1 (-190.0034, 10) -> (-190.0034, -10) centre (-190, 0) ccw
  line L1 (-190.0034, 10) -> (-160.0034, 10)
  circle A2 centre (-20.0339, 0) radius 4
  line L2 (-10, -15.0111) -> (-10, 15.0111)
  line L3 (-10, 15.0111) -> (-230, 15.0111)
  line L4 (-230, 15.0111) -> (-230, -15.0111)
  line L5 (-230, -15.0111) -> (-10, -15.0111)
  line L6 (0, 0) -> (-40, 0)
  line L7 (-40, 0) -> (-30, 0)
  line L8 (-30, 0) -> (-30, -12.5)
  line L9 (-30, -12.5) -> (-40, -12.5)
  line L10 (-40, -12.5) -> (-40, 0)
  line L11 (-40, 0) -> (-30, 0)
  line L12 (-30, 0) -> (-30, 12.5)
  line L13 (-30, 12.5) -> (-40, 12.5)
  line L14 (-40, 12.5) -> (-40, 0)
  dimension "d210" = 40
  dimension "d211" = 10
  dimension "d212" = 12.5
  dimension "d213" = 10
  dimension "d214" = 12.5
  constraint coincident L6.start origin
  constraint horizontal L6
  constraint horizontal L7
  constraint vertical L8
  constraint horizontal L9
  constraint vertical L10
  constraint horizontal L11
  constraint vertical L12
  constraint horizontal L13
  constraint vertical L14
  measures "d210" distance of L6.start L6.end
  measures "d211" distance of L6.end L7.end
  measures "d212" distance of L6.end L9.end
  measures "d213" distance of L6.end L7.end
  measures "d214" distance of L6.end L13.end
extrude "Estrusione50" add sketch "Schizzo87" along normal blind 26 separate body contours L6 L7 L8 L9 L10 L11 | L6 L7 L11 L12 L13 L14 picked at (-36.6667, -4.1667) picked at (-33.3333, 4.1667) makes body 15
sketch "Schizzo88" plane through (-1, 0, 0) normal (1, 0, 0) x (0, 0, -1)
  line L0 (7.2169, 12.5) -> (-7.2169, 12.5)
  line L1 (-7.2169, 12.5) -> (-14.4338, 0)
  line L2 (-14.4338, 0) -> (-7.2169, -12.5)
  line L3 (-7.2169, -12.5) -> (7.2169, -12.5)
  line L4 (7.2169, -12.5) -> (14.4338, 0)
  line L5 (14.4338, 0) -> (7.2169, 12.5)
  circle A0 centre (0, 0) radius 3.1
  line L6 (0, 0) -> (2, 0)
  line L7 (2, 0) -> (3.6508, 0)
  line L8 (3.6508, 0) -> (3.6508, 2.8801)
  line L9 (3.6508, 2.8801) -> (2, 2.8801)
  line L10 (2, 2.8801) -> (2, 0)
  line L11 (2, 0) -> (3.6508, 0)
  line L12 (3.6508, 0) -> (3.6508, -2.8167)
  line L13 (3.6508, -2.8167) -> (2, -2.8167)
  line L14 (2, -2.8167) -> (2, 0)
  dimension "d217" = 6.2
  dimension "d221" = 2
  constraint coincident A0.centre L6.start
  constraint horizontal L6
  constraint horizontal L7
  constraint vertical L8
  constraint horizontal L9
  constraint vertical L10
  constraint horizontal L11
  constraint vertical L12
  constraint horizontal L13
  constraint vertical L14
  measures "d217" diameter of A0
  measures "d221" distance of A0.centre L6.end
extrude "Estrusione51" cut sketch "Schizzo88" against normal blind 5 contours A0 L10 L14 picked at (-1.3945, 0) bodies 14
ref_plane "Piano di lavoro26" through (-6, 0, 1.133) normal (1, 0, 0) x (0, 0, -1)
sketch "Schizzo89" plane through (-6, 0, 0) normal (1, 0, 0) x (0, 0, -1)
ref_plane "Piano di lavoro27" through (-6, 0, 1.133) normal (1, 0, 0) x (0, 0, -1)
sketch "Schizzo90" plane through (-6, 0, 0) normal (1, 0, 0) x (0, 0, -1)
  circle A0 centre (0, 0) radius 3
  line L0 (0, 0) -> (2, 0)
  line L1 (2, 0) -> (3.4834, 0)
  line L2 (3.4834, 0) -> (3.4834, 2.8262)
  line L3 (3.4834, 2.8262) -> (2, 2.8262)
  line L4 (2, 2.8262) -> (2, 0)
  line L5 (2, 0) -> (3.4834, 0)
  line L6 (3.4834, 0) -> (3.4834, -2.8586)
  line L7 (3.4834, -2.8586) -> (2, -2.8586)
  line L8 (2, -2.8586) -> (2, 0)
  dimension "d223" = 6
  dimension "d224" = 2
  constraint coincident A0.centre L0.start
  constraint horizontal L0
  constraint horizontal L1
  constraint vertical L2
  constraint horizontal L3
  constraint vertical L4
  constraint horizontal L5
  constraint vertical L6
  constraint horizontal L7
  constraint vertical L8
  measures "d223" diameter of A0
  measures "d224" distance of A0.centre L0.end
extrude "Estrusione52" add sketch "Schizzo90" along normal blind 30 separate body contours A0 L4 L8 picked at (-1.3278, 0) makes body 16
sketch "Schizzo91" plane through (18, 9, -15.5885) normal (-0.707107, -0.353553, 0.612372) x (0.654654, 0, 0.755929)
  line L0 (-16.1481, -9.6214) -> (-4.8008, 18.1738)
  line L1 (-4.8008, 18.1738) -> (-15.7117, 28.8642)
  line L2 (-15.7117, 28.8642) -> (-31.4234, -9.6214)
  line L3 (-31.4234, -9.6214) -> (-16.1481, -9.6214)
sketch "Schizzo92" plane through (0, 0, 0) normal (0, 0, 1) x (1, 0, 0)
sketch "Schizzo93" plane through (24, 0, 0) normal (1, 0, 0) x (0, 0, -1)
  arc A0 (2, 2.2361) -> (2, -2.2361) centre (0, 0) ccw
  line L0 (2, -2.2361) -> (2, 2.2361)
  circle A1 centre (0, 0) radius 4
  dimension "d227" = 8
  constraint concentric A0 A1
  measures "d227" diameter of A1
extrude "Estrusione53" add sketch "Schizzo93" against normal blind 4 contours A1 picked at (2.6667, 0) bodies 16
ref_plane "Piano di lavoro28" through (10, 0, 0) normal (1, 0, 0) x (0, 0, -1)
sketch "Schizzo94" plane through (10, 0, 0) normal (1, 0, 0) x (0, 0, -1)
  circle A0 centre (0, 0) radius 5
  dimension "d231" = 10
  constraint coincident A0.centre origin
  measures "d231" diameter of A0
ref_plane "Piano di lavoro29" through (15, 0, 0) normal (1, 0, 0) x (0, 0, -1)
sketch "Schizzo95" plane through (15, 0, 0) normal (1, 0, 0) x (0, 0, -1)
  circle A0 centre (0, 0) radius 2
  dimension "d233" = 4
  constraint coincident A0.centre origin
  measures "d233" diameter of A0
loft "Loft5" add profiles "Schizzo94", "Schizzo95" section 1 contours A0 picked at (1.3101, -1.9935) section 2 contours A0 picked at (0.637, 0.1965) bodies 16
ref_plane "Piano di lavoro32" through (44, 0, 0) normal (1, 0, 0) x (0, 0, -1)
sketch "Schizzo98" plane through (44, 0, 0) normal (1, 0, 0) x (0, 0, -1)
  line L0 (0, 0) -> (0, 5)
  line L1 (0, 5) -> (25.9, 5)
  line L2 (25.9, 5) -> (25.9, 7)
  line L3 (25.9, 7) -> (0, 7)
  line L4 (0, 7) -> (0, 5)
  line L5 (25.9, 7) -> (20.0081, 17.2051)
  line L6 (25.9, 7) -> (37.6578, 7) construction
  line L7 (20.0081, 17.2051) -> (20.0081, 7)
  line L8 (20.0081, 7) -> (25.9, 7)
  dimension "d237" = 5
  dimension "d238" = 25.9
  dimension "d239" = 2
  dimension "d240" = 120
  constraint coincident L0.start origin
  constraint vertical L0
  constraint horizontal L1
  constraint vertical L2
  constraint horizontal L3
  constraint vertical L4
  constraint horizontal L6
  constraint perpendicular L3 L7
  constraint coincident L3 L7.end
  measures "d237" distance of L0.start L0.end
  measures "d238" distance of L0.end L1.end
  measures "d239" distance of L0.end L3.end
  measures "d240" angle of L5 L6
extrude "Estrusione54" add sketch "Schizzo98" along normal blind 140 separate body contours L1 L2 L3 L4 L8 | L3 L5 L7 L8 picked at (15.3027, 5.6667) picked at (21.972, 10.4017) makes body 17
copy_body "CopiaIncollaCorpi1" bodies 17 makes body 18
move_body "Sposta6" bodies 18 to x (-1, 0, 0) y (0, 1, 0) z (0, 0, -1) at (228, 0, 0)
combine "Combina1" operation add target body 17 tool bodies 18
move_body "Sposta7" bodies 17 to x (1, 0, 0) y (0, 1, 0) z (0, 0, 1) at (2, 0, 0)
ref_plane "Piano di lavoro33" through (20, 0, 0) normal (-1, 0, 0) x (0, 0, 1)
sketch "Schizzo99" plane through (20, 0, 0) normal (-1, 0, 0) x (0, 0, 1)
  circle A0 centre (0, 0) radius 4
  dimension "d244" = 8
  constraint coincident A0.centre origin
  measures "d244" diameter of A0
extrude "Estrusione55" add sketch "Schizzo99" along normal blind 9.5 contours A0 picked at (-1.2456, 0.0132) bodies 16
ref_plane "Piano di lavoro34" through (115, 18, -31.1769) normal (0, 0.5, -0.866025) x (0, -0.866025, -0.5)